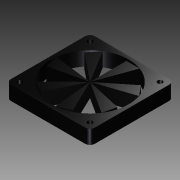
# Autodesk Inventor part: Fan60mm
Saved by Autodesk Inventor 2015 SP1 (Build 190203100, 203)
## iProperties
Created: 2014-02-07
Part Number: Fan60mm
Material: ABS Plastic
Document SubType Name: Modeling
Designer: Jack
Density: 1.06 g/cm^3
Appearance: Smooth - Black
Author: Jack
Autodesk Inventor part; units mm, degrees
ref_plane "YZ Plane" through (0, 0, 0) normal (1, 0, 0) x (0, 1, 0)
ref_plane "XZ Plane" through (0, 0, 0) normal (0, 1, 0) x (-1, 0, 0)
ref_plane "XY Plane" through (0, 0, 0) normal (0, 0, 1) x (1, 0, 0)
sketch "Sketch1" plane through (0, 0, 0) normal (0, 0, 1) x (1, 0, 0)
  line L0 (0, 0) -> (60, 0)
  line L1 (60, 0) -> (60, 60)
  line L2 (60, 60) -> (0, 60)
  line L3 (0, 60) -> (0, 0)
  dimension "d0" = 60
  dimension "d1" = 60
  constraints: 8 end point, 2 perpendicular, 1 horizontal, 1 parallel
  measures "d0" distance of L0.start L0.end
  measures "d1" distance of L0.end L1.end
extrude "Extrusion1" add sketch "Sketch1" along normal blind 10
hole "Hole1" at (5, 55, 10) direction (0, 0, -1) diameter 3.5 end through all
hole "Hole2" at (5, 5, 10) direction (0, 0, -1) diameter 3.5 end through all
hole "Hole3" at (55, 5, 10) direction (0, 0, -1) diameter 3.5 end through all
hole "Hole4" at (55, 55, 10) direction (0, 0, -1) diameter 3.5 end through all
fillet "Fillet1" radius 3.5 4 edges at (60, 0, 5) (0, 0, 5) (0, 60, 5) (60, 60, 5)
sketch "Sketch2" plane through (0, 0, 10) normal (0, 0, 1) x (1, 0, 0)
  line L0 (56.5, 60) -> (3.5, 60) projected
  line L1 (0, 56.5) -> (0, 3.5) projected
  line L2 (3.5, 0) -> (56.5, 0) projected
  line L3 (60, 3.5) -> (60, 56.5) projected
  line L4 (30, 60) -> (30, 0) construction
  line L5 (0, 30) -> (60, 30) construction
  line L6 (30, 30) -> (30, 56)
  line L7 (30, 30) -> (39.4632, 56)
  line L8 (39.4632, 56) -> (30, 56)
  line L9 (30, 30) -> (9.6724, 46.2107)
  line L10 (30, 30) -> (15.5726, 53.6094)
  line L11 (15.5726, 53.6094) -> (9.6724, 46.2107)
  line L12 (30, 30) -> (4.6519, 24.2145)
  line L13 (30, 30) -> (2.5461, 33.4404)
  line L14 (2.5461, 33.4404) -> (4.6519, 24.2145)
  line L15 (30, 30) -> (18.719, 6.5748)
  line L16 (30, 30) -> (10.193, 10.6807)
  line L17 (10.193, 10.6807) -> (18.719, 6.5748)
  line L18 (30, 30) -> (41.281, 6.5748)
  line L19 (30, 30) -> (32.7549, 2.4689)
  line L20 (32.7549, 2.4689) -> (41.281, 6.5748)
  line L21 (30, 30) -> (55.3481, 24.2145)
  line L22 (30, 30) -> (53.2424, 14.9885)
  line L23 (53.2424, 14.9885) -> (55.3481, 24.2145)
  line L24 (30, 30) -> (50.3276, 46.2107)
  line L25 (30, 30) -> (56.2278, 38.8121)
  line L26 (56.2278, 38.8121) -> (50.3276, 46.2107)
  circle A0 centre (30, 30) radius 27.6686
  point P0 (0, 0)
  dimension "d41" = 26
  dimension "d42" = 20
  dimension "d45" = 360
  constraints: 46 end point, 5 midpoint, 3 coincident, 1 perpendicular, 1 point on line, 44 other
  measures "d41" distance of L6.start L6.end
  measures "d42" angle of L7 L4
extrude "Extrusion2" cut sketch "Sketch2" against normal blind 10 contours L10 A0 L8 L6 | L13 A0 L11 L9 | L16 A0 L14 L12 | L19 A0 L17 L15 | L22 A0 L20 L18 | L25 A0 L23 L21 | L7 A0 L26 L24
body "Solid1"
